Autodesk Fusion 360 part; units mm, degrees
(part 6 of 6)
sketch "Sketch18" plane through (0, -8.5, 0) normal (0, 1, 0) x (-1, 0, 0)
  arc A0 (-137.9765, 39.7794) -> (-138.3203, 40.7036) centre (-138.2265, 40.2125) ccw
  arc A1 (-158.6031, 53.7396) -> (-138.3203, 40.7036) centre (-141.6031, 57.8929) ccw
  line L0 (-158.6031, 53.7396) -> (-158.6031, 62.0462)
  arc A2 (-125.0753, 63.6447) -> (-158.6031, 62.0462) centre (-141.6031, 57.8929) ccw
  arc A3 (-125.0753, 63.6447) -> (-124.1031, 63.809) centre (-124.6031, 63.809) ccw
  line L1 (-124.1031, 63.809) -> (-124.1031, 75.1805)
  arc A4 (-124.1031, 75.1805) -> (-161.7839, 71.9587) centre (-141.6031, 57.8929) ccw
  line L2 (-161.7839, 71.9587) -> (-161.7839, 43.8272)
  arc A5 (-161.7839, 43.8272) -> (-147.8246, 34.0937) centre (-141.6031, 57.8929) ccw
  line L3 (-147.8246, 34.0937) -> (-137.9765, 39.7794)
  circle A6 centre (-146.7556, 76.7997) radius 1.1
  circle A7 centre (-157.6917, 44.4147) radius 1.1
  circle A8 centre (-146.7556, 37.8883) radius 1.1
  circle A9 centre (-146.7556, 76.7997) radius 1.1
  circle A10 centre (-157.6917, 44.4147) radius 1.1
  circle A11 centre (-146.7556, 37.8883) radius 1.1
  arc A12 (-137.9765, 39.7794) -> (-138.3203, 40.7036) centre (-138.2265, 40.2125) ccw
  line L4 (-137.9765, 39.7794) -> (-147.8246, 34.0937)
  arc A13 (-161.7839, 43.8272) -> (-147.8246, 34.0937) centre (-141.6031, 57.8929) ccw
  line L5 (-161.7839, 43.8272) -> (-161.7839, 71.9587)
  arc A14 (-124.1031, 75.1805) -> (-161.7839, 71.9587) centre (-141.6031, 57.8929) ccw
  line L6 (-124.1031, 75.1805) -> (-124.1031, 63.809)
  arc A15 (-125.0753, 63.6447) -> (-124.1031, 63.809) centre (-124.6031, 63.809) ccw
  arc A16 (-125.0753, 63.6447) -> (-158.6031, 62.0462) centre (-141.6031, 57.8929) ccw
  line L7 (-158.6031, 62.0462) -> (-158.6031, 53.7396)
  arc A17 (-158.6031, 53.7396) -> (-138.3203, 40.7036) centre (-141.6031, 57.8929) ccw
  circle A18 centre (-141.6031, 57.8929) radius 16
  circle A19 centre (-141.6031, 57.8929) radius 17.5
  line L8 (-124.1031, 63.809) -> (-124.1031, 57.8929)
  line L9 (-137.9765, 39.7794) -> (-132.8531, 42.7375)
  line L10 (-141.6031, 57.8929) -> (-141.6031, 75.3929)
  line L11 (-141.6031, 57.8929) -> (-151.0058, 72.6523)
  line L12 (-141.6031, 57.8929) -> (-156.3624, 67.2957)
  circle A20 centre (-150.7371, 72.2306) radius 0.5
  circle A21 centre (-155.9407, 67.027) radius 0.5
  line L13 (-149.757, 71.6593) -> (-155.3695, 66.0468)
  line L14 (-150.7371, 72.2306) -> (-155.9407, 67.027)
  circle A22 centre (-150.7371, 72.2306) radius 0.75
  circle A23 centre (-155.9407, 67.027) radius 0.75
  circle A24 centre (-142.569, 57.6341) radius 15
  circle A25 centre (-141.3442, 58.8589) radius 15
  point P0 (-127.2654, 67.027)
  point P1 (-132.469, 72.2306)
  point P2 (-153.6239, 45.8721)
  dimension "d638" = 32
  dimension "d639" = 35
  dimension "d645" = 32.5
  dimension "d646" = 25
  dimension "d647" = 1
  dimension "d648" = 1
  dimension "d649" = 15.5
  dimension "d650" = 1.5
  dimension "d651" = 1.5
  dimension "d652" = 30
  dimension "d653" = 30
  constraint concentric A13 A18
  constraint concentric A13 A19
  constraint coincident A3.end L1.start
  constraint tangent A3 L8
  constraint parallel L6 L8
  constraint coincident A19 L8.end
  constraint coincident A0.start L3.end
  constraint tangent A0 L9
  constraint parallel L4 L9
  constraint coincident A19 L9.end
  constraint coincident A1.centre A2.centre
  constraint coincident A2 L10.end
  constraint parallel L1 L10
  constraint coincident A16 L11.end
  constraint coincident A2 L12.end
  constraint coincident L11 A20.centre
  constraint coincident L12 A21.centre
  constraint tangent A19 A20
  constraint tangent A19 A21
  constraint coincident A18 L13.start
  constraint coincident A18 L13.end
  constraint coincident A20.centre L14.start
  constraint coincident A21.centre L14.end
  constraint parallel L13 L14
  constraint concentric A20 A22
  constraint concentric A21 A23
  constraint tangent A18 A24
  constraint tangent L13 A24
  constraint tangent A18 A25
  constraint tangent L13 A25
  measures "d638" diameter of A18
  measures "d639" diameter of A19
  measures "d645" angle of L10 L11
  measures "d646" angle of L11 L12
  measures "d647" diameter of A20
  measures "d648" diameter of A21
  measures "d649" distance of A1.centre L13
  measures "d650" diameter of A22
  measures "d651" diameter of A23
  measures "d652" diameter of A24
  measures "d653" diameter of A25
extrude "Extrude13" add sketch "Sketch18" along normal blind 1.2 separate body contours A0 A1 A2 A3 L1 A4 L2 A5 L3 A12 L4 A13 L5 A14 L6 A15 A16 A17 A19 A22 A23 | A0 A12 A19 L9 | A1 L0 A2 A16 L7 A17 A18 A19 L10 L12 A23 | L0 L7 A19 | A3 A15 A19 L8 | A2 A16 A18 A19 L10 L11 A22 | A2 A16 A19 L14 A22 A23 | A18 L11 L12 L14 A22 A23 | A18 L10 L11 L13 A25 | A18 L12 L13 | A18 L11 L12 L13 | A18 L11 L13 | A18 L12 L13 A24 | L12 L13 A24 | L11 L13 A25 makes body 48
copy_body "Body->Comp4" bodies 47 removing the originals makes body 49 in component "cirque plate a"
copy_body "Body->Comp5" bodies 48 removing the originals makes body 50 in component "cirque plate b"
sketch "Sketch19" plane through (0, -9.7, 0) normal (0, -1, 0) x (1, 0, 0)
  circle A0 centre (146.7556, 76.7997) radius 1.1
  circle A1 centre (157.6917, 44.4147) radius 1.1
  circle A2 centre (146.7556, 37.8883) radius 1.1
  arc A3 (138.3203, 40.7036) -> (137.9765, 39.7794) centre (138.2265, 40.2125) ccw
  line L0 (137.9765, 39.7794) -> (147.8246, 34.0937)
  arc A4 (147.8246, 34.0937) -> (161.7839, 43.8272) centre (141.6031, 57.8929) ccw
  line L1 (161.7839, 43.8272) -> (161.7839, 71.9587)
  arc A5 (161.7839, 71.9587) -> (124.1031, 75.1805) centre (141.6031, 57.8929) ccw
  line L2 (124.1031, 75.1805) -> (124.1031, 63.809)
  arc A6 (124.1031, 63.809) -> (125.0753, 63.6447) centre (124.6031, 63.809) ccw
  arc A7 (158.6031, 62.0462) -> (125.0753, 63.6447) centre (141.6031, 57.8929) ccw
  line L3 (158.6031, 62.0462) -> (158.6031, 53.7396)
  arc A8 (138.3203, 40.7036) -> (158.6031, 53.7396) centre (141.6031, 57.8929) ccw
sketch "Sketch20" plane through (0, -9.7, 0) normal (0, -1, 0) x (1, 0, 0)
  line L0 (47.9031, 20.3158) -> (65.9031, 20.3158)
  line L1 (65.9031, 20.3158) -> (65.9031, 38.3158)
  line L2 (65.9031, 38.3158) -> (47.9031, 38.3158)
  line L3 (47.9031, 38.3158) -> (47.9031, 20.3158)
  line L4 (84.9531, 41.7294) -> (66.9531, 41.7294)
  line L5 (135.4448, 19.2441) -> (119.8563, 28.2441)
  line L6 (126.8413, 2.1738) -> (135.8413, 17.7623)
  line L7 (136.3663, 18.6838) -> (145.3663, 34.2723)
  line L8 (65.9031, 38.3158) -> (65.9031, 20.3158)
  line L9 (66.9531, 40.6794) -> (84.9531, 40.6794)
  line L10 (84.9531, 40.6794) -> (84.9531, 22.6794)
  line L11 (84.9531, 22.6794) -> (66.9531, 22.6794)
  line L12 (66.9531, 22.6794) -> (66.9531, 40.6794)
  line L13 (144.4448, 34.8326) -> (135.4448, 19.2441)
  line L14 (135.8413, 17.7623) -> (151.4298, 8.7623)
  line L15 (142.4298, -6.8262) -> (126.8413, 2.1738)
  line L16 (134.9023, 18.3044) -> (125.9023, 2.716)
  line L17 (134.9023, 18.3044) -> (119.3138, 27.3044)
  line L18 (125.9023, 2.716) -> (110.3138, 11.716)
  line L19 (110.3138, 11.716) -> (119.3138, 27.3044)
  line L20 (86.0031, 39.3658) -> (86.0031, 57.3658)
  line L21 (118.3798, 27.8437) -> (109.3798, 12.2552)
  line L22 (118.3798, 27.8437) -> (102.7914, 36.8437)
  line L23 (109.3798, 12.2552) -> (93.7914, 21.2552)
  line L24 (93.7914, 21.2552) -> (102.7914, 36.8437)
  dimension "d656" = 18
  dimension "d657" = 18
  dimension "d658" = 18
  dimension "d659" = 18
  dimension "d660" = 18
  dimension "d661" = 1.05
  dimension "d662" = 1.05
  dimension "d663" = 1.05
  dimension "d664" = 18
  dimension "d665" = 18
  dimension "d666" = 1.0785
  dimension "d667" = 1.0785
  constraint horizontal L9
  constraint vertical L10
  constraint horizontal L11
  constraint vertical L12
  constraint parallel L6 L16
  constraint collinear L13 L16
  constraint perpendicular L16 L17
  constraint collinear L14 L17
  constraint perpendicular L16 L18
  constraint perpendicular L18 L19
  constraint parallel L19 L21
  constraint perpendicular L21 L22
  constraint collinear L17 L22
  constraint perpendicular L21 L23
  constraint perpendicular L23 L24
  measures "d656" distance of L1.end L0.end
  measures "d657" distance of L16.start L16.end
  measures "d658" distance of L16.start L17.end
  measures "d659" distance of L10.end L11.end
  measures "d660" distance of L9.start L11.end
  measures "d661" distance of L4.start L20
  measures "d662" distance of L8 L12
  measures "d663" distance of L4.start L9.end
  measures "d664" distance of L21.start L21.end
  measures "d665" distance of L21.start L22.end
  measures "d666" distance of L5.start L7.start
  measures "d667" distance of L19 L21
extrude "Extrude14" add sketch "Sketch20" against normal up to surface (4 mm away) separate body contours L9 L10 L11 L12 | L16 L17 L18 L19 | L21 L22 L23 L24 makes body 51 at (72.9531, -9.7, 34.6794) makes body 52 at (101.9875, -9.7, 23.4514) makes body 53 at (126.7061, -9.7, 16.1083)
ref_plane "WorkPlane5" through (155.7839, 9, 98.4665) normal (0, 0, 1) x (0, 1, 0)
sketch "Sketch21" plane through (0, 0, 98.4665) normal (0, 0, 1) x (1, 0, 0)
  line L0 (153.2839, 11.8) -> (158.2839, 11.8)
  line L1 (155.7839, 3.4) -> (155.7839, 14.6)
  line L2 (161.3465, 14.975) -> (161.3465, 16.325)
  line L3 (161.3465, 14.975) -> (155.7839, 14.975)
  line L4 (156.3465, 21.325) -> (155.7839, 21.325)
  line L5 (155.7839, 21.325) -> (155.7839, 14.6)
  line L6 (157.5365, 14.975) -> (157.5365, 11.8)
  arc A0 (161.3465, 16.325) -> (156.3465, 21.325) centre (156.3465, 16.325) ccw
  line L7 (156.3465, 16.325) -> (161.3465, 16.325)
  line L8 (156.3465, 16.325) -> (156.3465, 21.325)
  dimension "d671" = 1.7526
  dimension "d672" = 5.5626
  dimension "d673" = 5
  dimension "d674" = 6.35
  dimension "d698" = 3.175
  constraint vertical L2
  constraint coincident L1 L3.end
  constraint perpendicular L1 L3
  constraint perpendicular L1 L4
  constraint coincident L1.end L5.end
  constraint perpendicular L4 L5
  constraint coincident L3 L6.start
  constraint coincident L0 L6.end
  constraint perpendicular L0 L6
  constraint coincident A0.centre L7.start
  constraint horizontal L7
  constraint perpendicular L7 L8
  constraint coincident L4.start A0
  constraint coincident L4.start A0.end
  constraint coincident L2.end A0.start
  measures "d671" distance of L1 L6
  measures "d672" distance of L1 L2
  measures "d673" distance of L2.end A0.centre
  measures "d674" distance of L3 L4
  measures "d698" distance of L3 L6.end
revolve "Revolve1" add sketch "Sketch21" angle 360 about axis through (155.7839, 3.4, 98.4665) along (0, 1, 0) separate body makes body 54
copy_body "Body->Comp6" bodies 54 removing the originals makes body 55 in component "foot"
sketch "Sketch22" plane through (0, 2.5, 0) normal (0, -1, 0) x (1, 0, 0)
  line L0 (103.8578, 14.9931) -> (142.6281, -7.5847)
  line L1 (142.6281, -7.5847) -> (161.7839, 25.5411)
  line L2 (161.7839, 25.5411) -> (161.7839, 103.1522)
  line L3 (161.7839, 103.1522) -> (123.6486, 112.6772)
  line L4 (123.6486, 112.6772) -> (84.9842, 117.4397)
  line L5 (84.9842, 117.4397) -> (66.9572, 117.4397)
  line L6 (66.9572, 117.4397) -> (9.2428, 110.3136)
  line L7 (9.2428, 110.3136) -> (9.2428, 14.9931)
  line L8 (9.2428, 14.9931) -> (103.8578, 14.9931)
  line L9 (142.1031, 84.5919) -> (142.1031, 102.5919)
  line L10 (142.1031, 102.5919) -> (124.1031, 102.5919)
  line L11 (124.1031, 102.5919) -> (124.1031, 84.5919)
  line L12 (124.1031, 84.5919) -> (142.1031, 84.5919)
  line L13 (123.0531, 93.0669) -> (123.0531, 75.0669)
  line L14 (142.1031, 93.5919) -> (143.1531, 93.5919)
  line L15 (143.1531, 93.5919) -> (152.1531, 93.5919)
  circle A0 centre (152.1531, 93.5919) radius 6.5
  dimension "d677" = 1.05
  dimension "d678" = 1.05
  dimension "d679" = 18
  dimension "d680" = 9
  dimension "d681" = 13
  constraint midpoint L9 L14.start
  constraint perpendicular L9 L14
  constraint horizontal L15
  constraint coincident L15.end A0.centre
  measures "d677" distance of L11 L13.start
  measures "d678" distance of L14.start L14.end
  measures "d679" distance of L9.end L10.end
  measures "d680" distance of L14.end L15.end
  measures "d681" diameter of A0
extrude "Extrude15" add sketch "Sketch22" along normal blind 13 from surface at 9.5 separate body contours A0 makes body 56
sketch "Sketch23" plane through (0, -9.7, 0) normal (0, -1, 0) x (1, 0, 0)
  arc A0 (158.6031, 62.0462) -> (125.0753, 63.6447) centre (141.6031, 57.8929) ccw
  circle A1 centre (141.6031, 57.8929) radius 17.5
  dimension "d685" = 35
  constraint concentric A0 A1
  measures "d685" diameter of A1
extrude "Extrude16" add sketch "Sketch23" along normal blind 0.2 separate body makes body 57
extrude "Extrude17" add sketch "top plate" along normal blind 1.2 separate body contours L0 L1 L2 L3 L4 A0 A1 A2 A3 A4 A5 A6 L5 L6 L7 L8 L9 L10 L11 L12 L145 L147 A18 L157 A19 L159 makes body 58
sketch "Sketch24" plane through (0, 2.5, 0) normal (0, -1, 0) x (1, 0, 0)
  line L0 (103.8578, 14.9931) -> (142.6281, -7.5847)
  line L1 (142.6281, -7.5847) -> (161.7839, 25.5411)
  line L2 (161.7839, 25.5411) -> (161.7839, 103.1522)
  line L3 (161.7839, 103.1522) -> (123.6486, 112.6772)
  line L4 (123.6486, 112.6772) -> (84.9842, 117.4397)
  line L5 (84.9842, 117.4397) -> (66.9572, 117.4397)
  line L6 (66.9572, 117.4397) -> (9.2428, 110.3136)
  line L7 (9.2428, 110.3136) -> (9.2428, 14.9931)
  line L8 (9.2428, 14.9931) -> (103.8578, 14.9931)
  line L9 (142.1031, 46.4919) -> (142.1031, 64.4919)
  line L10 (142.1031, 64.4919) -> (124.1031, 64.4919)
  line L11 (124.1031, 64.4919) -> (124.1031, 46.4919)
  line L12 (124.1031, 46.4919) -> (142.1031, 46.4919)
  line L13 (123.0531, 54.9669) -> (123.0531, 36.9669)
  line L14 (142.1031, 55.4919) -> (143.1531, 55.4919)
  line L15 (143.1531, 55.4919) -> (152.1531, 55.4919)
  circle A0 centre (152.1531, 55.4919) radius 6.5
  dimension "d690" = 1.05
  dimension "d691" = 18
  dimension "d692" = 1.05
  dimension "d693" = 9
  dimension "d694" = 13
  constraint midpoint L9 L14.start
  constraint perpendicular L9 L14
  constraint perpendicular L9 L15
  constraint coincident L15.end A0.centre
  measures "d690" distance of L11 L13.start
  measures "d691" distance of L9.end L10.end
  measures "d692" distance of L14.start L14.end
  measures "d693" distance of L14.end L15.end
  measures "d694" diameter of A0
extrude "Extrude18" add sketch "Sketch24" along normal up to surface (13 mm away) from surface at 9.5 separate body contours A0 makes body 59
ref_plane "WorkPlane6" through (155.7839, 9, 27.151) normal (0, 0, 1) x (0, 1, 0)
sketch "Sketch25" plane through (0, 0, 27.151) normal (0, 0, 1) x (1, 0, 0)
  line L0 (155.7839, 21.325) -> (155.7839, 14.1092)
  line L1 (157.5365, 14.975) -> (157.5365, 11.8)
  line L2 (161.3465, 14.975) -> (161.3465, 16.325)
  line L3 (161.3465, 14.975) -> (155.7839, 14.975)
  arc A0 (161.3465, 16.325) -> (156.3465, 21.325) centre (156.3465, 16.325) ccw
  line L4 (156.3465, 16.325) -> (156.3465, 21.325)
  line L5 (156.3465, 16.325) -> (161.3465, 16.325)
  line L6 (156.3465, 21.325) -> (155.7839, 21.325)
  line L7 (155.7839, 2.9092) -> (155.7839, 14.1092)
  line L8 (153.2839, 11.8) -> (158.2839, 11.8)
  line L9 (158.2839, 6.2) -> (153.2839, 6.2)
  line L10 (155.7839, 3.4) -> (155.7839, 14.6)
  point P0 (158.2839, 12.8)
  dimension "d700" = 1.7526
  dimension "d701" = 5.5626
  dimension "d702" = 5
  dimension "d703" = 6.35
  dimension "d704" = 3.175
  constraint vertical L2
  constraint coincident L3.end L7
  constraint perpendicular L3 L7
  constraint perpendicular L6 L7
  constraint coincident L0.end L7.end
  constraint perpendicular L0 L6
  constraint coincident L1.start L3
  constraint coincident A0.centre L4.start
  constraint horizontal L5
  constraint perpendicular L4 L5
  constraint coincident L4.end A0
  constraint coincident A0.end L4.end
  constraint coincident L2.end A0.start
  constraint coincident L1.end L8
  constraint collinear L7 L10
  measures "d700" distance of L1 L7
  measures "d701" distance of L2 L7
  measures "d702" distance of A0.centre L2.end
  measures "d703" distance of L3 L6
  measures "d704" distance of L1.end L3
revolve "Revolve2" add sketch "Sketch25" angle 360 about axis through (155.7839, 2.9092, 27.151) along (0, 1, 0) separate body makes body 60
ref_plane "WorkPlane7" through (97.1443, 9, -74.3275) normal (0, 0, 1) x (0, 1, 0)
sketch "Sketch26" plane through (0, 0, -74.3275) normal (0, 0, 1) x (1, 0, 0)
  line L0 (97.1443, 21.325) -> (97.1443, 14.6)
  line L1 (98.8969, 14.975) -> (98.8969, 11.8)
  line L2 (102.7069, 14.975) -> (102.7069, 16.325)
  line L3 (102.7069, 14.975) -> (97.1443, 14.975)
  arc A0 (102.7069, 16.325) -> (97.7069, 21.325) centre (97.7069, 16.325) ccw
  line L4 (97.7069, 16.325) -> (97.7069, 21.325)
  line L5 (97.7069, 16.325) -> (102.7069, 16.325)
  line L6 (97.7069, 21.325) -> (97.1443, 21.325)
  line L7 (97.1443, 3.4) -> (97.1443, 14.6)
  line L8 (97.1443, 3.4) -> (97.1443, 14.6)
  line L9 (94.6443, 11.8) -> (99.6443, 11.8)
  point P0 (103.2839, 26.8)
  dimension "d707" = 1.7526
  dimension "d708" = 5.5626
  dimension "d709" = 5
  dimension "d710" = 6.35
  dimension "d711" = 3.175
  constraint vertical L2
  constraint coincident L3.end L7
  constraint perpendicular L3 L7
  constraint perpendicular L6 L7
  constraint coincident L0.end L7.end
  constraint perpendicular L0 L6
  constraint coincident L1.start L3
  constraint coincident A0.centre L4.start
  constraint horizontal L5
  constraint perpendicular L4 L5
  constraint coincident L4.end A0
  constraint coincident A0.end L4.end
  constraint coincident L2.end A0.start
  constraint collinear L7 L8
  constraint coincident L1.end L9
  measures "d707" distance of L1 L7
  measures "d708" distance of L2 L7
  measures "d709" distance of A0.centre L2.end
  measures "d710" distance of L3 L6
  measures "d711" distance of L1.end L3
revolve "Revolve3" add sketch "Sketch26" angle 360 about axis through (97.1443, 3.4, -74.3275) along (0, 1, 0) separate body makes body 61
ref_plane "WorkPlane8" through (15.2428, 9, -74.3275) normal (0, 0, 1) x (0, 1, 0)
sketch "Sketch27" plane through (0, 0, -74.3275) normal (0, 0, 1) x (1, 0, 0)
  line L0 (15.2428, 21.325) -> (15.2428, 14.6)
  line L1 (16.9954, 14.975) -> (16.9954, 11.8)
  line L2 (20.8054, 14.975) -> (20.8054, 16.325)
  line L3 (20.8054, 14.975) -> (15.2428, 14.975)
  arc A0 (20.8054, 16.325) -> (15.8054, 21.325) centre (15.8054, 16.325) ccw
  line L4 (15.8054, 16.325) -> (15.8054, 21.325)
  line L5 (15.8054, 16.325) -> (20.8054, 16.325)
  line L6 (15.8054, 21.325) -> (15.2428, 21.325)
  line L7 (15.2428, 3.4) -> (15.2428, 14.6)
  line L8 (15.2428, 3.4) -> (15.2428, 14.6)
  line L9 (12.7428, 11.8) -> (17.7428, 11.8)
  point P0 (18.2839, 31.8)
  dimension "d714" = 1.7526
  dimension "d715" = 5.5626
  dimension "d716" = 5
  dimension "d717" = 6.35
  dimension "d718" = 3.175
  constraint vertical L2
  constraint coincident L3.end L7
  constraint perpendicular L3 L7
  constraint perpendicular L6 L7
  constraint coincident L0.end L7.end
  constraint perpendicular L0 L6
  constraint coincident L1.start L3
  constraint coincident A0.centre L4.start
  constraint horizontal L5
  constraint perpendicular L4 L5
  constraint coincident L4.end A0
  constraint coincident A0.end L4.end
  constraint coincident L2.end A0.start
  constraint collinear L7 L8
  constraint coincident L1.end L9
  measures "d714" distance of L1 L7
  measures "d715" distance of L2 L7
  measures "d716" distance of A0.centre L2.end
  measures "d717" distance of L3 L6
  measures "d718" distance of L1.end L3
revolve "Revolve4" add sketch "Sketch27" angle 360 about axis through (15.2428, 3.4, -74.3275) along (0, 1, 0) separate body makes body 62
ref_plane "WorkPlane9" through (15.2428, 9, 105.0089) normal (0, 0, 1) x (0, 1, 0)
sketch "Sketch28" plane through (0, 0, 105.0089) normal (0, 0, 1) x (1, 0, 0)
  line L0 (15.2428, 21.325) -> (15.2428, 14.6)
  line L1 (16.9954, 14.975) -> (16.9954, 11.8)
  line L2 (20.8054, 14.975) -> (20.8054, 16.325)
  line L3 (20.8054, 14.975) -> (15.2428, 14.975)
  arc A0 (20.8054, 16.325) -> (15.8054, 21.325) centre (15.8054, 16.325) ccw
  line L4 (15.8054, 16.325) -> (15.8054, 21.325)
  line L5 (15.8054, 16.325) -> (20.8054, 16.325)
  line L6 (15.8054, 21.325) -> (15.2428, 21.325)
  line L7 (15.2428, 3.4) -> (15.2428, 14.6)
  line L8 (15.2428, 3.4) -> (15.2428, 14.6)
  line L9 (12.7428, 11.8) -> (17.7428, 11.8)
  point P0 (23.2839, 31.8)
  dimension "d721" = 1.7526
  dimension "d722" = 5.5626
  dimension "d723" = 5
  dimension "d724" = 6.35
  dimension "d725" = 3.175
  constraint vertical L2
  constraint coincident L3.end L7
  constraint perpendicular L3 L7
  constraint perpendicular L6 L7
  constraint coincident L0.end L7.end
  constraint perpendicular L0 L6
  constraint coincident L1.start L3
  constraint coincident A0.centre L4.start
  constraint horizontal L5
  constraint perpendicular L4 L5
  constraint coincident L4.end A0
  constraint coincident A0.end L4.end
  constraint coincident L2.end A0.start
  constraint collinear L7 L8
  constraint coincident L1.end L9
  measures "d721" distance of L1 L7
  measures "d722" distance of L2 L7
  measures "d723" distance of A0.centre L2.end
  measures "d724" distance of L3 L6
  measures "d725" distance of L1.end L3
revolve "Revolve5" add sketch "Sketch28" angle 360 about axis through (15.2428, 3.4, 105.0089) along (0, 1, 0) separate body makes body 63
copy_body "Body->Comp7" bodies 43 removing the originals makes body 64 in component "wrist rest"
extrude "Extrude12" [suppressed]
component "top plate" placed x (1, 0, 0) y (0, 1, 0) z (0, 0, 1) at (0, 0, 0)
component "baseplate" placed x (1, 0, 0) y (0, 1, 0) z (0, 0, 1) at (0, 0, 0)
component "battery plate" placed x (1, 0, 0) y (0, 1, 0) z (0, 0, 1) at (0, 0, 0)
component "top plate" placed x (1, 0, 0) y (0, 1, 0) z (0, 0, 1) at (0, 0, 0)
component "cirque plate a" placed x (1, 0, 0) y (0, 1, 0) z (0, 0, 1) at (0, 0, 0)
component "cirque plate b" placed x (1, 0, 0) y (0, 1, 0) z (0, 0, 1) at (0, 0, 0)
component "foot" placed x (1, 0, 0) y (0, 1, 0) z (0, 0, 1) at (0, 0, 0)
component "wrist rest" placed x (1, 0, 0) y (0, 1, 0) z (0, 0, 1) at (0, 0, 0)
hidden bodies 51 52 53 57
equation "d17 = d16"
equation "d57 = d56"
equation "d59 = d58"
equation "d60 = d59 / 2"
equation "d61 = d60"
equation "d62 = d58 + d60"
equation "d63 = d62"
equation "d77 = d76"
equation "d82 = d81"
equation "d83 = d82 / 2"
equation "d84 = d81 + d83"
equation "d89 = d88"
equation "d90 = d89"
equation "d92 = d91"
equation "d93 = d58"
equation "d94 = d58"
equation "d98 = d97"
equation "d100 = d99"
equation "d101 = d102"
equation "d103 = d102 * 2"
equation "d106 = d104"
equation "d107 = d104"
equation "d108 = d106"
equation "d109 = d104"
equation "d110 = d104"
equation "d111 = d102"
equation "d112 = d102"
equation "d113 = d111"
equation "d114 = d111"
equation "d116 = d115"
equation "d117 = d111"
equation "d272 = d271"
equation "d282 = d281"
equation "d286 = d285 / 2"
equation "d287 = d284 / 2"
equation "d288 = d285"
equation "d289 = d288 / 2"
equation "d291 = d290 / 2"
equation "d292 = d290"
equation "d293 = d291"
equation "d296 = d294 / 2"
equation "d297 = d296"
equation "d298 = d282"
equation "d299 = d282"
equation "d329 = d328"
equation "d331 = d330"
equation "d440 = d436"
equation "d441 = d436"
equation "d454 = d436"
equation "d455 = d436"
equation "d468 = d436"
equation "d469 = d436"
equation "d484 = d436"
equation "d485 = d436"
equation "d500 = d436"
equation "d501 = d436"
equation "d516 = d436"
equation "d517 = d436"
equation "d532 = d436"
equation "d533 = d436"
equation "d545 = d549"
equation "d585 = 1.05 mm * 2"
equation "d589 = d588"
equation "d590 = d588"
equation "d597 = d595"
equation "d598 = d595"
equation "d599 = d596"
equation "d600 = d596"
equation "d621 = d620 / 2"
equation "d629 = d626"
equation "d631 = d630"
equation "d633 = 135 deg + 32.5 deg"
equation "d649 = ( 31 / 2 ) * 1 mm"
equation "d657 = d656"
equation "d658 = d656"
equation "d659 = d656"
equation "d660 = d656"
equation "d662 = d661"
equation "d663 = d661"
equation "d664 = d659"
equation "d665 = d659"
equation "d667 = d666"
equation "d671 = 0.138 in / 2"
equation "d672 = 0.438 in / 2"
equation "d678 = d677"
equation "d680 = d679 / 2"
equation "d682 = 5 mm + 4.5 mm"
equation "d692 = d690"
equation "d693 = d691 / 2"
equation "d698 = 0.25 in / 2"
equation "d700 = 0.138 in / 2"
equation "d701 = 0.438 in / 2"
equation "d704 = 0.25 in / 2"
equation "d707 = 0.138 in / 2"
equation "d708 = 0.438 in / 2"
equation "d711 = 0.25 in / 2"
equation "d714 = 0.138 in / 2"
equation "d715 = 0.438 in / 2"
equation "d718 = 0.25 in / 2"
equation "d721 = 0.138 in / 2"
equation "d722 = 0.438 in / 2"
equation "d725 = 0.25 in / 2"
named bodies: "top plate", "pcb", "nn adapter", "baseplate", "battery", "mock nn", "battery plate", "wrist rest"
